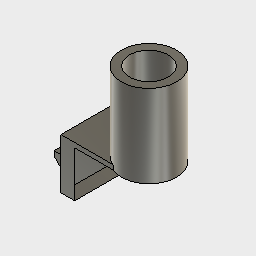
Adam - Y Rod Holder UNFINISHED (Autodesk Fusion 360 design; units mm, degrees)
Autodesk Fusion 360 part; units mm, degrees
cylinder "CylinderPrimitive1" add diameter 12 height 18 placed x (1, 0, 0) y (0, 1, 0) z (0, 0, 1) at (0, 0, 0) makes body 1
copy_body "CutPasteBodies1" bodies 1 body 1 seen with x (0, 0, 0) y (0, 0, 0) z (0, 0, 0) at (0, 0, 0) removing the originals makes body 2 in component "Component"
hole "Hole1" at (0, 0, 18) direction (0, 0, -1) diameter 8.4 depth 15 tip angle 118 bodies 2 in component "Component"
sketch "Sketch1" plane through (0, 0, 0) normal (0, 0, 1) x (1, 0, 0) in component "Component"
sketch "Sketch2" plane through (0, 0, 0) normal (0, 0, -1) x (1, 0, 0) in component "Component"
  circle A0 centre (0, 0) radius 6
  line L0 (-2.2798, -5.55) -> (-2.2798, 5.55)
  line L1 (-2.2798, 5.55) -> (-13.6398, 5.55)
  line L2 (-13.6398, 5.55) -> (-13.6398, -5.55)
  line L3 (-13.6398, -5.55) -> (-2.2798, -5.55)
  line L4 (-10.6398, -5.55) -> (-10.6398, 5.55)
  dimension "d6" = 11.1
  dimension "d7" = 11.36
  dimension "d8" = 3
  constraint coincident A0
  constraint vertical L0
  constraint perpendicular L0 L1
  constraint perpendicular L1 L2
  constraint perpendicular L0 L3
  constraint coincident L3
  constraint coincident L1
  constraint perpendicular L1 L4
  measures "d8" distance of L2 L4
extrude "Extrude1" add sketch "Sketch2" against normal blind 1 contours A0 L1 L3 L4 | L1 L2 L3 L4 bodies 2 in component "Component"
sketch "Sketch3" plane through (0, -5.55, 0) normal (0, -1, 0) x (1, 0, 0) in component "Component"
  line L0 (-13.6398, 0) -> (-2.2798, 0)
  line L1 (-2.2798, 0) -> (-2.2798, 1)
  line L2 (-2.2798, 1) -> (-13.6398, 1)
  line L3 (-13.6398, 1) -> (-13.6398, 0)
  line L4 (-13.6398, 1) -> (-13.6398, -10)
  line L5 (-13.6398, -10) -> (-10.6398, -10)
  line L6 (-10.6398, -10) -> (-10.6398, 1)
  dimension "d11" = 11
  dimension "d12" = 3
  constraint perpendicular L0 L4
  constraint perpendicular L5 L6
extrude "Extrude2" add sketch "Sketch3" against normal up to surface (11.1 mm away) contours L0 L4 L5 L6 bodies 2 in component "Component"
sketch "Sketch4" plane through (0, -5.55, 0) normal (0, -1, 0) x (1, 0, 0) in component "Component"
  line L0 (-10.6398, 0) -> (-2.2798, 0)
  line L1 (-2.2798, 0) -> (-2.2798, 1)
  line L2 (-2.2798, 1) -> (-13.6398, 1)
  line L3 (-13.6398, 1) -> (-13.6398, -10)
  line L4 (-13.6398, -10) -> (-10.6398, -10)
  line L5 (-10.6398, -10) -> (-10.6398, 0)
  line L6 (-13.6398, -10) -> (-10.6398, -10)
  line L7 (-2.2798, 1) -> (-2.2798, 0)
  line L8 (-10.6398, -7) -> (-3.6398, 0)
  dimension "d14" = 3
  dimension "d15" = 1.36
  constraint coincident L5
  constraint coincident L0
extrude "Extrude3" add sketch "Sketch4" against normal blind 1.5 separate body contours L0 L5 L8 makes body 3 in component "Component"
ref_plane "WorkPlane1" through (-7.9598, 0, -4.5) normal (0, 1, 0) x (-1, 0, 0) in component "Component"
mirror "Mirror1" about plane through (-7.9598, 0, -4.5) normal (0, 1, 0) of bodies 3 makes body 4 in component "Component"
sketch "Sketch5" plane through (-13.6398, 0, 0) normal (-1, 0, 0) x (0, -1, 0) in component "Component"
  line L0 (5.55, -10) -> (5.55, 1)
  line L1 (5.55, 1) -> (-5.55, 1)
  line L2 (-5.55, 1) -> (-5.55, -10)
  line L3 (-5.55, -10) -> (5.55, -10)
  circle A0 centre (0, -4.5) radius 1.6
  dimension "d19" = 3.2
  dimension "d20" = 5.55
  dimension "d21" = 5.5
  measures "d19" diameter of A0
  measures "d20" distance of L0
  measures "d21" distance of L1
extrude "Extrude4" cut sketch "Sketch5" against normal up to surface (3 mm away) contours A0 bodies 2 in component "Component"
sketch "Sketch6" plane through (0, 5.55, 0) normal (0, 1, 0) x (-1, 0, 0) in component "Component"
  line L0 (13.6398, -10) -> (13.6398, 1)
  line L1 (13.6398, 1) -> (2.2798, 1)
  line L2 (2.2798, 1) -> (2.2798, 0)
  line L3 (2.2798, 0) -> (10.6398, 0)
  line L4 (10.6398, 0) -> (10.6398, -10)
  line L5 (10.6398, -10) -> (13.6398, -10)
  line L6 (13.6398, -2.8) -> (15.1398, -2.8)
  line L7 (15.1398, -2.8) -> (15.1398, -3.8)
  line L8 (15.1398, -3.8) -> (13.6398, -5.3)
  line L9 (15.1398, -3.8) -> (13.6398, -3.8) construction
  dimension "d23" = 1.5
  dimension "d24" = 1
  dimension "d25" = 1.5
  dimension "d26" = 3.8
  constraint coincident L0
  constraint perpendicular L0 L6
  constraint perpendicular L6 L7
  constraint perpendicular L0 L9
  measures "d26" distance of L1
extrude "Extrude5" add sketch "Sketch6" against normal blind 1.5 separate body contours L0 L6 L7 L8 makes body 5 in component "Component"
mirror "Mirror2" about plane through (-7.9598, 0, -4.5) normal (0, 1, 0) of bodies 5 makes body 6 in component "Component"
component "Component" placed x (1, 0, 0) y (0, 1, 0) z (0, 0, 1) at (0, 0, 0)
equation "d20 = 3.95 mm + 1.60 mm"
